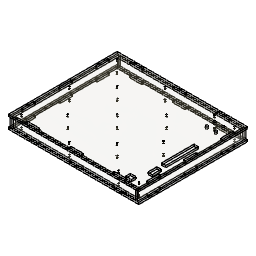
enclosure (Autodesk Fusion 360 design; units mm, degrees)
Autodesk Fusion 360 part; units mm, degrees
note: some values were not read from the file. Set by a fixed rule: which sketch regions a step uses.
sketch "Sketch1" plane through (157.5, -130, 0) normal (0, 0, 1) x (1, 0, 0) in component "Bottom_Plate"
  circle A0 centre (95, 77.5) radius 1.1
  circle A1 centre (62.5, 77.5) radius 1.1
  circle A2 centre (-95, 77.5) radius 1.1
  circle A3 centre (-17.5, 77.5) radius 1.1
  circle A4 centre (22.5, 40) radius 1.1
  circle A5 centre (-57.5, 40) radius 1.1
  circle A6 centre (-95, 0) radius 1.1
  circle A7 centre (-17.5, 0) radius 1.1
  circle A8 centre (57.5, 0) radius 1.1
  circle A9 centre (-57.5, -40) radius 1.1
  circle A10 centre (22.5, -40) radius 1.1
  circle A11 centre (-95, -77.5) radius 1.1
  circle A12 centre (-17.5, -77.5) radius 1.1
  circle A13 centre (62.5, -77.5) radius 1.1
  circle A14 centre (95, -77.5) radius 1.1
  line L0 (105.5, -88) -> (-105.5, -88)
  line L1 (-105.5, -88) -> (-105.5, 88)
  line L2 (-105.5, 88) -> (62.5, 88)
  line L3 (62.5, 88) -> (77.5, 88)
  line L4 (77.5, 88) -> (105.5, 88)
  line L5 (105.5, 88) -> (105.5, -88)
  line L6 (0, 88) -> (0, -88) construction
  line L7 (105.5, 0) -> (-105.5, 0) construction
  line L8 (70, 88) -> (70, -88) construction
  line L9 (105.5, 60) -> (-105.5, 60) construction
  line L10 (60, 85.5) -> (80, 85.5)
  line L11 (80, 85.5) -> (80, 82.5)
  line L12 (80, 82.5) -> (60, 82.5)
  line L13 (60, 82.5) -> (60, 85.5)
  line L14 (-70, 88) -> (-70, -88) construction
  line L15 (-60, 85.5) -> (-80, 85.5)
  line L16 (-60, 82.5) -> (-60, 85.5)
  line L17 (-80, 82.5) -> (-60, 82.5)
  line L18 (-80, 85.5) -> (-80, 82.5)
  line L19 (-60, -85.5) -> (-80, -85.5)
  line L20 (-80, -82.5) -> (-60, -82.5)
  line L21 (-80, -85.5) -> (-80, -82.5)
  line L22 (-60, -82.5) -> (-60, -85.5)
  line L23 (60, -85.5) -> (80, -85.5)
  line L24 (60, -82.5) -> (60, -85.5)
  line L25 (80, -82.5) -> (60, -82.5)
  line L26 (80, -85.5) -> (80, -82.5)
  line L27 (100, 70) -> (103, 70)
  line L28 (103, 70) -> (103, 50)
  line L29 (103, 50) -> (100, 50)
  line L30 (100, 50) -> (100, 70)
  line L31 (100, -50) -> (100, -70)
  line L32 (100, -70) -> (103, -70)
  line L33 (103, -70) -> (103, -50)
  line L34 (103, -50) -> (100, -50)
  line L35 (105.5, -60) -> (-105.5, -60) construction
  line L36 (-100, 50) -> (-100, 70)
  line L37 (-100, 70) -> (-103, 70)
  line L38 (-103, 70) -> (-103, 50)
  line L39 (-103, 50) -> (-100, 50)
  line L40 (-103, -50) -> (-100, -50)
  line L41 (-100, -50) -> (-100, -70)
  line L42 (-103, -70) -> (-103, -50)
  line L43 (-100, -70) -> (-103, -70)
  line L44 (-10, 85.5) -> (10, 85.5)
  line L45 (10, 85.5) -> (10, 82.5)
  line L46 (10, 82.5) -> (-10, 82.5)
  line L47 (-10, 82.5) -> (-10, 85.5)
  line L48 (-10, -85.5) -> (10, -85.5)
  line L49 (-10, -82.5) -> (-10, -85.5)
  line L50 (10, -82.5) -> (-10, -82.5)
  line L51 (10, -85.5) -> (10, -82.5)
  line L52 (100, 10) -> (103, 10)
  line L53 (103, 10) -> (103, -10)
  line L54 (103, -10) -> (100, -10)
  line L55 (100, -10) -> (100, 10)
  line L56 (-100, -10) -> (-100, 10)
  line L57 (-100, 10) -> (-103, 10)
  line L58 (-103, 10) -> (-103, -10)
  line L59 (-103, -10) -> (-100, -10)
  circle A15 centre (-95, 77.5) radius 1.1
  circle A16 centre (-95, 77.5) radius 1.1
  circle A17 centre (-17.5, 77.5) radius 1.1
  circle A18 centre (-17.5, 77.5) radius 1.1
  circle A19 centre (62.5, 77.5) radius 1.1
  circle A20 centre (95, 77.5) radius 1.1
  circle A21 centre (-57.5, 40) radius 1.1
  circle A22 centre (-57.5, 40) radius 1.1
  circle A23 centre (22.5, 40) radius 1.1
  circle A24 centre (-95, 0) radius 1.1
  circle A25 centre (-57.5, -40) radius 1.1
  circle A26 centre (-95, -77.5) radius 1.1
  circle A27 centre (-17.5, 0) radius 1.1
  circle A28 centre (57.5, 0) radius 1.1
  circle A29 centre (22.5, -40) radius 1.1
  circle A30 centre (-17.5, -77.5) radius 1.1
  circle A31 centre (62.5, -77.5) radius 1.1
  circle A32 centre (95, -77.5) radius 1.1
  dimension "d6" = 70
  dimension "d7" = 60
  dimension "d10" = 20
  dimension "d11" = 3
  dimension "d13" = 10
  dimension "d15" = 3
  dimension "d16" = 20
  dimension "d18" = 2.5
  dimension "d19" = 2.5
  dimension "d20" = 10
  dimension "d21" = 20
  dimension "d22" = 3
  dimension "d24" = 10
  dimension "d25" = 2.5
  dimension "d26" = 3
  dimension "d27" = 20
  dimension "d28" = 10
  dimension "d29" = 2.5
  dimension "d30" = 2.2
  dimension "d31" = 2.2
  dimension "d32" = 2.2
  dimension "d33" = 2.2
  dimension "d34" = 2.2
  dimension "d35" = 2.2
  dimension "d36" = 2.2
  dimension "d37" = 2.2
  dimension "d39" = 2.2
  dimension "d40" = 2.2
  dimension "d41" = 2.2
  dimension "d42" = 2.2
  dimension "d43" = 2.2
  dimension "d44" = 2.2
  dimension "d45" = 2.2
  constraint coincident L2 L6.start
  constraint midpoint L0 L6.end
  constraint perpendicular L0 L6
  constraint midpoint L5 L7.start
  constraint midpoint L1 L7.end
  constraint coincident L2 L8.start
  constraint coincident L0 L8.end
  constraint perpendicular L0 L8
  constraint coincident L5 L9.start
  constraint coincident L1 L9.end
  constraint perpendicular L1 L9
  constraint horizontal L10
  constraint vertical L11
  constraint horizontal L12
  constraint vertical L13
  constraint symmetric L6 L8.start L14.start
  constraint symmetric L6 L8.end L14.end
  constraint symmetric L6 L10.start L15.start
  constraint symmetric L6 L10.end L15.end
  constraint symmetric L6 L11.end L17.start
  constraint symmetric L6 L12.end L16.start
  constraint symmetric L7 L10.start L23.start
  constraint symmetric L7 L10.end L23.end
  constraint symmetric L7 L11.end L25.start
  constraint symmetric L7 L12.end L24.start
  constraint symmetric L7 L15.start L19.start
  constraint symmetric L7 L15.end L19.end
  constraint symmetric L7 L16.start L20.end
  constraint symmetric L7 L17.start L20.start
  constraint horizontal L27
  constraint vertical L28
  constraint horizontal L29
  constraint vertical L30
  constraint symmetric L7 L9.start L35.start
  constraint symmetric L7 L9.end L35.end
  constraint symmetric L7 L27.start L31.end
  constraint symmetric L7 L27.end L32.end
  constraint symmetric L7 L28.end L33.end
  constraint symmetric L7 L29.end L31.start
  constraint symmetric L6 L27.start L36.end
  constraint symmetric L6 L27.end L37.end
  constraint symmetric L6 L28.end L38.end
  constraint symmetric L6 L29.end L36.start
  constraint symmetric L6 L31.start L40.end
  constraint symmetric L6 L31.end L41.end
  constraint symmetric L6 L32.end L42.start
  constraint symmetric L6 L33.end L40.start
  constraint horizontal L44
  constraint vertical L45
  constraint horizontal L46
  constraint vertical L47
  constraint symmetric L7 L44.start L48.start
  constraint symmetric L7 L44.end L48.end
  constraint symmetric L7 L45.end L50.start
  constraint symmetric L7 L46.end L49.start
  constraint horizontal L52
  constraint vertical L53
  constraint horizontal L54
  constraint vertical L55
  constraint symmetric L6 L52.start L56.end
  constraint symmetric L6 L52.end L57.end
  constraint symmetric L6 L53.end L58.end
  constraint symmetric L6 L54.end L56.start
  constraint concentric A2 A15
  constraint concentric A15 A16
  constraint concentric A3 A17
  constraint concentric A17 A18
  constraint concentric A1 A19
  constraint concentric A0 A20
  constraint concentric A5 A21
  constraint concentric A5 A22
  constraint concentric A4 A23
  constraint concentric A6 A24
  constraint concentric A9 A25
  constraint concentric A11 A26
  constraint concentric A7 A27
  constraint concentric A8 A28
  constraint concentric A10 A29
  constraint concentric A12 A30
  constraint concentric A13 A31
  constraint concentric A14 A32
  measures "d6" distance of L6 L8
  measures "d7" distance of L7 L9
  measures "d10" distance of L10.start L10.end
  measures "d11" distance of L10.start L12.end
  measures "d13" distance of L8 L11
  measures "d15" distance of L27.start L27.end
  measures "d16" distance of L27.end L28.end
  measures "d18" distance of L4 L10
  measures "d19" distance of L5 L28
  measures "d20" distance of L9 L27
  measures "d21" distance of L44.start L44.end
  measures "d22" distance of L44.start L46.end
  measures "d24" distance of L6 L45
  measures "d25" distance of L2 L44
  measures "d26" distance of L52.start L52.end
  measures "d27" distance of L52.start L54.end
  measures "d28" distance of L7 L52
  measures "d29" distance of L5 L53
  measures "d30" diameter of A16
  measures "d31" diameter of A18
  measures "d32" diameter of A19
  measures "d33" diameter of A20
  measures "d34" diameter of A22
  measures "d35" diameter of A23
  measures "d36" diameter of A24
  measures "d37" diameter of A25
  measures "d39" diameter of A26
  measures "d40" diameter of A27
  measures "d41" diameter of A28
  measures "d42" diameter of A29
  measures "d43" diameter of A30
  measures "d44" diameter of A31
  measures "d45" diameter of A32
extrude "Extrude1" add sketch "Sketch1" along normal blind 3 makes body 1 in component "Bottom_Plate"
ref_plane "WorkPlane1" through (105.5, 88, 18) normal (0, 0, 1) x (1, 0, 0) in component "Top_Plate"
sketch "Sketch1 (2)" plane through (105.5, 88, 18) normal (0, 0, 1) x (1, 0, 0) in component "Top_Plate"
  line L0 (80, 85.5) -> (80, 82.5)
  line L1 (60, 85.5) -> (80, 85.5)
  line L2 (60, 82.5) -> (60, 85.5)
  line L3 (80, 82.5) -> (60, 82.5)
  circle A0 centre (95, -77.5) radius 1.1
  circle A1 centre (62.5, -77.5) radius 1.1
  circle A2 centre (-17.5, -77.5) radius 1.1
  circle A3 centre (22.5, -40) radius 1.1
  circle A4 centre (57.5, 0) radius 1.1
  circle A5 centre (-17.5, 0) radius 1.1
  circle A6 centre (-95, -77.5) radius 1.1
  circle A7 centre (-57.5, -40) radius 1.1
  circle A8 centre (-95, 0) radius 1.1
  circle A9 centre (22.5, 40) radius 1.1
  circle A10 centre (-57.5, 40) radius 1.1
  circle A11 centre (95, 77.5) radius 1.1
  circle A12 centre (-95, 77.5) radius 1.1
  circle A13 centre (-17.5, 77.5) radius 1.1
  line L4 (-100, 10) -> (-100, -10)
  line L5 (-103, 10) -> (-100, 10)
  line L6 (-103, -10) -> (-103, 10)
  line L7 (-100, -10) -> (-103, -10)
  circle A14 centre (62.5, 77.5) radius 1.1
  line L8 (103, 10) -> (103, -10)
  line L9 (100, 10) -> (103, 10)
  line L10 (100, -10) -> (100, 10)
  line L11 (103, -10) -> (100, -10)
  line L12 (-10, -82.5) -> (10, -82.5)
  line L13 (-10, -85.5) -> (-10, -82.5)
  line L14 (10, -85.5) -> (-10, -85.5)
  line L15 (10, -82.5) -> (10, -85.5)
  line L16 (10, 85.5) -> (10, 82.5)
  line L17 (-10, 85.5) -> (10, 85.5)
  line L18 (-10, 82.5) -> (-10, 85.5)
  line L19 (10, 82.5) -> (-10, 82.5)
  line L20 (-103, -50) -> (-100, -50)
  line L21 (-103, -70) -> (-103, -50)
  line L22 (-100, -70) -> (-103, -70)
  line L23 (-100, -50) -> (-100, -70)
  line L24 (-100, 70) -> (-100, 50)
  line L25 (-103, 70) -> (-100, 70)
  line L26 (-103, 50) -> (-103, 70)
  line L27 (-100, 50) -> (-103, 50)
  line L28 (100, -70) -> (100, -50)
  line L29 (103, -70) -> (100, -70)
  line L30 (103, -50) -> (103, -70)
  line L31 (100, -50) -> (103, -50)
  line L32 (-60, 82.5) -> (-80, 82.5)
  line L33 (-60, 85.5) -> (-60, 82.5)
  line L34 (-80, 85.5) -> (-60, 85.5)
  line L35 (-80, 82.5) -> (-80, 85.5)
  line L36 (-80, -85.5) -> (-80, -82.5)
  line L37 (-60, -85.5) -> (-80, -85.5)
  line L38 (-60, -82.5) -> (-60, -85.5)
  line L39 (-80, -82.5) -> (-60, -82.5)
  line L40 (60, -82.5) -> (80, -82.5)
  line L41 (60, -85.5) -> (60, -82.5)
  line L42 (80, -85.5) -> (60, -85.5)
  line L43 (80, -82.5) -> (80, -85.5)
  line L44 (103, 70) -> (103, 50)
  line L45 (100, 70) -> (103, 70)
  line L46 (100, 50) -> (100, 70)
  line L47 (103, 50) -> (100, 50)
  line L48 (105.5, 88) -> (105.5, -88)
  line L49 (105.5, -88) -> (-105.5, -88)
  line L50 (-105.5, -88) -> (-105.5, 88)
  line L51 (-105.5, 88) -> (105.5, 88)
extrude "Extrude1'" add sketch "Sketch1 (2)" along normal blind 3 separate body makes body 2 in component "Top_Plate"
sketch "Sketch1 (3)" plane through (5.5, 0, 0) normal (-1, 0, 0) x (0, -1, 0) in component "Side_1A"
  line L0 (-138, 18) -> (-138, 21)
  line L1 (-138, 21) -> (-158, 21)
  line L2 (-158, 21) -> (-158, 18)
  line L3 (-158, 18) -> (-158, 21)
  line L4 (-158, 21) -> (-138, 21)
  line L5 (-98, 18) -> (-98, 21)
  line L6 (-98, 21) -> (-78, 21)
  line L7 (-38, 18) -> (-38, 21)
  line L8 (-38, 21) -> (-18, 21)
  line L9 (-138, 18) -> (-138, 21)
  line L10 (-78, 18) -> (-78, 21)
  line L11 (-18, 18) -> (-18, 21)
  line L12 (-138, 0) -> (-138, 3)
  line L13 (-158, 0) -> (-138, 0)
  line L14 (-78, 0) -> (-78, 3)
  line L15 (-98, 0) -> (-78, 0)
  line L16 (-18, 0) -> (-18, 3)
  line L17 (-38, 0) -> (-18, 0)
  line L18 (-38, 0) -> (-38, 3)
  line L19 (-158, 0) -> (-158, 3)
  line L20 (-98, 0) -> (-98, 3)
  line L21 (-176, 18) -> (-176, 21)
  line L22 (-176, 0) -> (-176, 3)
  line L23 (0, 18) -> (0, 21)
  line L24 (0, 0) -> (0, 3)
  line L25 (-158, 18) -> (-176, 18)
  line L26 (-176, 3) -> (-158, 3)
  line L27 (-176, 18) -> (-176, 3)
  line L28 (-138, 3) -> (-137, 3)
  line L29 (-137, 3) -> (-98, 3)
  line L30 (-98, 18) -> (-138, 18)
  line L31 (-78, 18) -> (-38, 18)
  line L32 (-38, 3) -> (-78, 3)
  line L33 (-18, 18) -> (0, 18)
  line L34 (0, 18) -> (0, 3)
  line L35 (-18, 3) -> (0, 3)
  constraint coincident L2.end L3.start
  constraint coincident L21.start L25.end
  constraint coincident L22.end L26.start
  constraint coincident L19.end L26.end
  constraint coincident L12.end L28.start
  constraint perpendicular L12 L28
  constraint coincident L20.end L29.end
  constraint perpendicular L20 L29
  constraint coincident L5.start L30.start
  constraint coincident L0.start L9.start
  constraint coincident L10.start L31.start
  constraint coincident L7.start L31.end
  constraint coincident L18.end L32.start
  constraint coincident L14.end L32.end
  constraint coincident L11.start L33.start
  constraint coincident L23.start L33.end
  constraint coincident L24.end L34.end
  constraint coincident L16.end L35.start
extrude "Extrude1''" add sketch "Sketch1 (3)" along normal blind 3 separate body makes body 3 in component "Side_1A"
sketch "Sketch1 (4)" plane through (205.5, 0, 0) normal (1, 0, 0) x (0, 1, 0) in component "Side_1B"
  line L0 (98, 18) -> (98, 21)
  line L1 (98, 21) -> (78, 21)
  line L2 (78, 21) -> (78, 18)
  line L3 (38, 3) -> (38, 0)
  line L4 (78, 3) -> (38, 3)
  line L5 (78, 0) -> (78, 3)
  line L6 (98, 0) -> (78, 0)
  line L7 (98, 3) -> (98, 0)
  line L8 (138, 3) -> (98, 3)
  line L9 (138, 0) -> (138, 3)
  line L10 (158, 0) -> (138, 0)
  line L11 (158, 3) -> (158, 0)
  line L12 (176, 3) -> (158, 3)
  line L13 (176, 18) -> (176, 3)
  line L14 (158, 18) -> (176, 18)
  line L15 (158, 21) -> (158, 18)
  line L16 (138, 21) -> (158, 21)
  line L17 (138, 18) -> (138, 21)
  line L18 (98, 18) -> (138, 18)
  line L19 (98, 21) -> (98, 18)
  line L20 (78, 21) -> (98, 21)
  line L21 (78, 18) -> (78, 21)
  line L22 (38, 18) -> (78, 18)
  line L23 (38, 21) -> (38, 18)
  line L24 (18, 21) -> (38, 21)
  line L25 (18, 18) -> (18, 21)
  line L26 (0, 18) -> (18, 18)
  line L27 (0, 3) -> (0, 18)
  line L28 (18, 3) -> (0, 3)
  line L29 (18, 0) -> (18, 3)
  line L30 (38, 0) -> (18, 0)
extrude "Extrude1'''" add sketch "Sketch1 (4)" along normal blind 3 separate body makes body 4 in component "Side_1B"
sketch "Sketch1 (5)" plane through (0, 2.5, 0) normal (0, 1, 0) x (-1, 0, 0) in component "Side_2A"
  line L0 (-165.5, 18) -> (-165.5, 21)
  line L1 (-165.5, 21) -> (-185.5, 21)
  line L2 (-185.5, 21) -> (-185.5, 18)
  line L3 (-115.5, 21) -> (-95.5, 21)
  line L4 (-95.5, 18) -> (-95.5, 21)
  line L5 (-185.5, 21) -> (-165.5, 21)
  line L6 (-165.5, 18) -> (-165.5, 21)
  line L7 (-45.5, 21) -> (-25.5, 21)
  line L8 (-25.5, 18) -> (-25.5, 21)
  line L9 (-185.5, 18) -> (-185.5, 21)
  line L10 (-115.5, 18) -> (-115.5, 21)
  line L11 (-45.5, 18) -> (-45.5, 21)
  line L12 (-185.5, 0) -> (-165.5, 0)
  line L13 (-185.5, 0) -> (-185.5, 3)
  line L14 (-45.5, 0) -> (-25.5, 0)
  line L15 (-45.5, 0) -> (-45.5, 3)
  line L16 (-115.5, 0) -> (-95.5, 0)
  line L17 (-115.5, 0) -> (-115.5, 3)
  line L18 (-165.5, 0) -> (-165.5, 3)
  line L19 (-95.5, 0) -> (-95.5, 3)
  line L20 (-25.5, 0) -> (-25.5, 3)
  line L21 (-5.5, 18) -> (-5.5, 3)
  line L22 (-205.5, 3) -> (-205.5, 18)
  line L23 (-205.5, 18) -> (-185.5, 18)
  line L24 (-165.5, 18) -> (-115.5, 18)
  line L25 (-115.5, 3) -> (-165.5, 3)
  line L26 (-185.5, 3) -> (-205.5, 3)
  line L27 (-45.5, 18) -> (-95.5, 18)
  line L28 (-95.5, 3) -> (-45.5, 3)
  line L29 (-5.5, 18) -> (-25.5, 18)
  line L30 (-25.5, 3) -> (-5.5, 3)
  constraint coincident L22.end L23.start
  constraint coincident L2.end L9.start
  constraint coincident L0.start L6.start
  constraint coincident L10.start L24.end
  constraint coincident L17.end L25.start
  constraint coincident L18.end L25.end
  constraint coincident L13.end L26.start
  constraint coincident L22.start L26.end
  constraint coincident L11.start L27.start
  constraint coincident L4.start L27.end
  constraint coincident L19.end L28.start
  constraint coincident L15.end L28.end
  constraint coincident L21.start L29.start
  constraint coincident L8.start L29.end
  constraint coincident L20.end L30.start
  constraint coincident L21.end L30.end
extrude "Extrude1''''" add sketch "Sketch1 (5)" along normal blind 3 separate body makes body 5 in component "Side_2A"
sketch "Sketch1 (6)" plane through (0, 170.5, 0) normal (0, 1, 0) x (-1, 0, 0) in component "Side_2B"
  line L0 (-165.5, 18) -> (-165.5, 21)
  line L1 (-165.5, 21) -> (-185.5, 21)
  line L2 (-185.5, 21) -> (-185.5, 18)
  line L3 (-45.5, 0) -> (-45.5, 3)
  line L4 (-95.5, 3) -> (-45.5, 3)
  line L5 (-95.5, 0) -> (-95.5, 3)
  line L6 (-115.5, 0) -> (-95.5, 0)
  line L7 (-115.5, 0) -> (-115.5, 3)
  line L8 (-115.5, 3) -> (-165.5, 3)
  line L9 (-165.5, 0) -> (-165.5, 3)
  line L10 (-185.5, 0) -> (-165.5, 0)
  line L11 (-185.5, 0) -> (-185.5, 3)
  line L12 (-185.5, 3) -> (-205.5, 3)
  line L13 (-205.5, 3) -> (-205.5, 18)
  line L14 (-205.5, 18) -> (-185.5, 18)
  line L15 (-185.5, 18) -> (-185.5, 21)
  line L16 (-185.5, 21) -> (-165.5, 21)
  line L17 (-165.5, 18) -> (-165.5, 21)
  line L18 (-165.5, 18) -> (-115.5, 18)
  line L19 (-115.5, 18) -> (-115.5, 21)
  line L20 (-115.5, 21) -> (-95.5, 21)
  line L21 (-95.5, 18) -> (-95.5, 21)
  line L22 (-45.5, 18) -> (-95.5, 18)
  line L23 (-45.5, 18) -> (-45.5, 21)
  line L24 (-45.5, 21) -> (-25.5, 21)
  line L25 (-25.5, 18) -> (-25.5, 21)
  line L26 (-5.5, 18) -> (-25.5, 18)
  line L27 (-5.5, 18) -> (-5.5, 3)
  line L28 (-25.5, 3) -> (-5.5, 3)
  line L29 (-25.5, 0) -> (-25.5, 3)
  line L30 (-45.5, 0) -> (-25.5, 0)
extrude "Extrude1'''''" add sketch "Sketch1 (6)" along normal blind 3 separate body makes body 6 in component "Side_2B"
sketch "Sketch4" plane through (0, 0, 21) normal (0, 0, 1) x (-1, 0, 0) in component "Top_Plate"
  circle A0 centre (-10.5, -88) radius 1.1
  circle A1 centre (-200.5, -165.5) radius 1.1
  circle A2 centre (-10.5, -165.5) radius 1.1
  circle A3 centre (-128, -128) radius 1.1
  circle A4 centre (-48, -128) radius 1.1
  line L0 (-165.5, -5.5) -> (-185.5, -5.5)
  line L1 (-185.5, -5.5) -> (-185.5, -2.5)
  line L2 (-185.5, -2.5) -> (-165.5, -2.5)
  line L3 (-165.5, -2.5) -> (-165.5, -5.5)
  circle A5 centre (-128, -48) radius 1.1
  line L4 (-185.5, -173.5) -> (-185.5, -170.5)
  line L5 (-185.5, -170.5) -> (-165.5, -170.5)
  line L6 (-165.5, -170.5) -> (-165.5, -173.5)
  line L7 (-165.5, -173.5) -> (-185.5, -173.5)
  circle A6 centre (-163, -88) radius 1.1
  circle A7 centre (-168, -10.5) radius 1.1
  circle A8 centre (-48, -48) radius 1.1
  line L8 (-45.5, -170.5) -> (-25.5, -170.5)
  line L9 (-25.5, -170.5) -> (-25.5, -173.5)
  line L10 (-25.5, -173.5) -> (-45.5, -173.5)
  line L11 (-45.5, -173.5) -> (-45.5, -170.5)
  circle A9 centre (-10.5, -10.5) radius 1.1
  circle A10 centre (-88, -88) radius 1.1
  line L12 (-25.5, -2.5) -> (-25.5, -5.5)
  line L13 (-25.5, -5.5) -> (-45.5, -5.5)
  line L14 (-45.5, -5.5) -> (-45.5, -2.5)
  line L15 (-45.5, -2.5) -> (-25.5, -2.5)
  circle A11 centre (-88, -10.5) radius 1.1
  line L16 (-208.5, -158) -> (-208.5, -138)
  line L17 (-208.5, -138) -> (-205.5, -138)
  line L18 (-205.5, -138) -> (-205.5, -158)
  line L19 (-205.5, -158) -> (-208.5, -158)
  line L20 (-5.5, -98) -> (-5.5, -78)
  line L21 (-5.5, -78) -> (-2.5, -78)
  line L22 (-2.5, -78) -> (-2.5, -98)
  line L23 (-2.5, -98) -> (-5.5, -98)
  circle A12 centre (-88, -165.5) radius 1.1
  circle A13 centre (-200.5, -10.5) radius 1.1
  line L24 (-5.5, -158) -> (-5.5, -138)
  line L25 (-5.5, -138) -> (-2.5, -138)
  line L26 (-2.5, -138) -> (-2.5, -158)
  line L27 (-2.5, -158) -> (-5.5, -158)
  line L28 (-2.5, -38) -> (-5.5, -38)
  line L29 (-5.5, -38) -> (-5.5, -18)
  line L30 (-5.5, -18) -> (-2.5, -18)
  line L31 (-2.5, -18) -> (-2.5, -38)
  line L32 (-115.5, -173.5) -> (-115.5, -170.5)
  line L33 (-115.5, -170.5) -> (-95.5, -170.5)
  line L34 (-95.5, -170.5) -> (-95.5, -173.5)
  line L35 (-95.5, -173.5) -> (-115.5, -173.5)
  line L36 (-205.5, -18) -> (-205.5, -38)
  line L37 (-205.5, -38) -> (-208.5, -38)
  line L38 (-208.5, -38) -> (-208.5, -18)
  line L39 (-208.5, -18) -> (-205.5, -18)
  circle A14 centre (-168, -165.5) radius 1.1
  line L40 (-95.5, -5.5) -> (-115.5, -5.5)
  line L41 (-115.5, -5.5) -> (-115.5, -2.5)
  line L42 (-115.5, -2.5) -> (-95.5, -2.5)
  line L43 (-95.5, -2.5) -> (-95.5, -5.5)
  line L44 (-208.5, -98) -> (-208.5, -78)
  line L45 (-208.5, -78) -> (-205.5, -78)
  line L46 (-205.5, -78) -> (-205.5, -98)
  line L47 (-205.5, -98) -> (-208.5, -98)
  line L48 (0, -176) -> (0, 0)
  line L49 (0, 0) -> (-211, 0)
  line L50 (-211, 0) -> (-211, -176)
  line L51 (-211, -176) -> (0, -176)
  circle A15 centre (-177, -157.15) radius 2
  circle A16 centre (-191.25, -157.15) radius 2
  circle A17 centre (-177, -144.4) radius 2
  circle A18 centre (-191.25, -144.4) radius 2
  line L52 (-199.27, -55.47) -> (-199.27, -108.27)
  line L53 (-199.27, -108.27) -> (-192.19, -108.27)
  line L54 (-192.19, -108.27) -> (-192.19, -55.47)
  line L55 (-192.19, -55.47) -> (-199.27, -55.47)
  line L56 (-201.02, -31.82) -> (-201.02, -46.52)
  line L57 (-201.02, -46.52) -> (-193.94, -46.52)
  line L58 (-193.94, -46.52) -> (-193.94, -31.82)
  line L59 (-193.94, -31.82) -> (-201.02, -31.82)
  line L60 (-181.75, -12.9) -> (-181.75, -8)
  line L61 (-181.75, -8) -> (-191.15, -8)
  line L62 (-191.15, -8) -> (-191.15, -12.9)
  line L63 (-184.7, -15.75) -> (-181.75, -15.75)
  line L64 (-181.75, -15.75) -> (-181.75, -13.9)
  line L65 (-191.15, -13.9) -> (-191.15, -15.75)
  line L66 (-191.15, -15.75) -> (-188.2, -15.75)
  line L67 (-188.2, -15.75) -> (-184.7, -15.75)
  line L68 (-181.75, -13.9) -> (-181.75, -12.9)
  line L69 (-191.15, -13.9) -> (-191.15, -12.9)
  dimension "d57" = 4
  dimension "d58" = 4
  dimension "d59" = 4
  dimension "d60" = 4
  constraint parallel L63 L67
  constraint perpendicular L67 L68
  measures "d57" diameter of A15
  measures "d58" diameter of A16
  measures "d59" diameter of A17
  measures "d60" diameter of A18
extrude "Extrude2" cut sketch "Sketch4" against normal up to surface (3 mm away) contours A15 | A16 | A17 | A18 | L52 L53 L54 L55 | L56 L57 L58 L59 | L60 L61 L62 L63 L64 L65 L66 L67 L68 L69 bodies 2 in component "Top_Plate"
component "Bottom_Plate" placed x (1, 0, 0) y (0, 1, 0) z (0, 0, 1) at (-52, 218, 0)
component "Top_Plate" placed x (1, 0, 0) y (0, 1, 0) z (0, 0, 1) at (0, 0, 0)
component "Side_1A" placed x (1, 0, 0) y (0, 1, 0) z (0, 0, 1) at (0, 0, 0)
component "Side_1B" placed x (1, 0, 0) y (0, 1, 0) z (0, 0, 1) at (0, 0, 0)
component "Side_2A" placed x (1, 0, 0) y (0, 1, 0) z (0, 0, 1) at (0, 0, 0)
component "Side_2B" placed x (1, 0, 0) y (0, 1, 0) z (0, 0, 1) at (0, 0, 0)
equation "thickness = 3 mm"
equation "d3 = thickness"
equation "tabWidth = thickness"
equation "tabLength = 20 mm"
equation "d10 = tabLength"
equation "d11 = tabWidth"
equation "d13 = tabLength / 2"
equation "d15 = tabWidth"
equation "d16 = tabLength"
equation "d20 = tabLength / 2"
equation "d21 = tabLength"
equation "d22 = tabWidth"
equation "d24 = tabLength / 2"
equation "d26 = tabWidth"
equation "d27 = tabLength"
equation "d28 = tabLength / 2"
equation "d47 = thickness"
equation "d49 = thickness"
equation "d51 = thickness"
equation "d53 = thickness"
equation "d55 = thickness"
